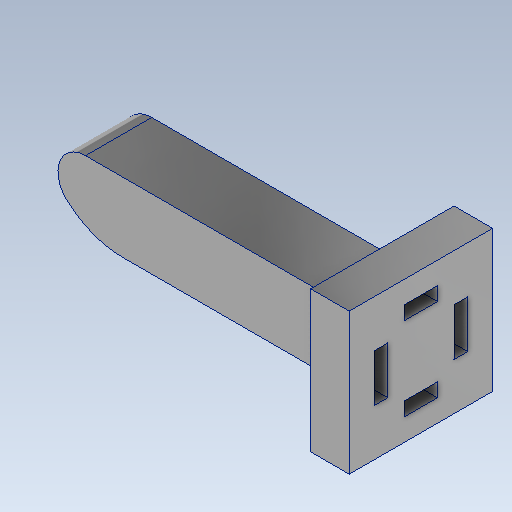
# Autodesk Inventor part: Finray_9_Kerbe_10deg_anschluss_erweitert_9_75 Nut
Saved by Autodesk Inventor 2025.2 (Build 292293000, 293)
## iProperties
Created: 2022-02-28
Part Number: Finray_9_Kerbe_10deg_anschluss_erweitert_9_75 Nut
Material: Generic
Document SubType Name: Modeling
Designer: richa
Density: 1 g/cm^3
Appearance: Aluminum - Flat
Author: richa
## iProperties of the stored document Maria_Greifer_3D-Druck.ipt
Created: 2024-11-10
Part Number: Maria_Greifer_3D-Druck
Material: Generisch
Document SubType Name: Modeling
Designer: maria
Density: 1 g/cm^3
Appearance: Vorgabe
Author: maria
Autodesk Inventor part; units mm, degrees
ref_plane "YZ Plane" through (0, 0, 0) normal (1, 0, 0) x (0, 1, 0)
ref_plane "XZ Plane" through (0, 0, 0) normal (0, 1, 0) x (-1, 0, 0)
ref_plane "XY Plane" through (0, 0, 0) normal (0, 0, 1) x (1, 0, 0)
sketch "Sketch5" plane through (0, 0, 0) normal (0, 0, 1) x (1, 0, 0)
  line L0 (48.5, 0) -> (3.8, 0)
  line L1 (48.5, -12.6) -> (3.8, -12.6)
  line L2 (3.8, -12.6) -> (0, -12.6)
  line L3 (0, -12.6) -> (0, 0)
  line L4 (0, 0) -> (7.8, 0)
  line L5 (38.5, 0) -> (38.5, -12.6)
  line L6 (37.5, -12.6) -> (37.5, 0)
  line L7 (0, -45.1294) -> (0, -34.3361)
  line L8 (0, -34.3361) -> (38.5, -34.3361)
  line L9 (38.5, -34.3361) -> (38.5, -45.1294)
  line L10 (38.5, -45.1294) -> (0, -45.1294)
  line L11 (38.5, -42.4105) -> (39.5, -42.4105)
  line L12 (39.5, -42.4105) -> (39.5, -38.1261)
  line L13 (39.5, -38.1261) -> (38.5, -38.1261)
  line L14 (39.5, -42.4105) -> (39.5, -49.5786)
  line L15 (39.5, -49.5786) -> (45, -49.5786)
  line L16 (45, -49.5786) -> (45, -34.3361)
  line L17 (45, -34.3361) -> (39.5, -34.3361)
  line L18 (39.5, -34.3361) -> (39.5, -38.1261)
  line L19 (48.5, 0) -> (55.8897, 0)
  line L20 (55.8897, 0) -> (55.8897, -12.6)
  line L21 (55.8897, -12.6) -> (48.5, -12.6)
  point P0 (7.8, 0)
  point P1 (39, -42.4105)
  dimension "d63" = 44.7
  dimension "d71" = 0
  dimension "d97" = 12.6
  dimension "d123" = 1
  dimension "d124" = 37.5
  dimension "d125" = 38.5
  dimension "d127" = 1
  dimension "d128" = 5.5
  constraints: 44 end point, 13 perpendicular, 8 point on line, 4 horizontal, 2 vertical, 1 midpoint, 1 parallel
  measures "d63" distance of L1.start L1.end
  measures "d71" distance from line of L3.end L0
  measures "d97" distance of L2.end L3.end
  measures "d123" distance between parallel lines of L5 L6
  measures "d124" distance between parallel lines of L3 L6
  measures "d125" distance of L9.end L7.start
  measures "d127" distance of L11.start L11.end
  measures "d128" distance of L14.end L15.end
extrude "Extrusion2" add sketch "Sketch5" along normal blind 12 contours L19 L20 L21 L1 L5 L0 | L5 L1 L6 L0 | L6 L1 L2 L3 L4 L0
fillet "Fillet2" radius 15 1 edges at (0, -12.6, 6)
fillet "Rundung3" radius 5 1 edges at (0, 0, 6)
sketch "Skizze17" plane through (55.8897, -12.6, 0) normal (1, 0, 0) x (0, 0, -1)
  line L0 (-19, -6.5) -> (7, -6.5)
  line L1 (7, -6.5) -> (7, 19.1)
  line L2 (7, 19.1) -> (-19, 19.1)
  line L3 (-19, 19.1) -> (-19, -6.5)
  line L4 (-19, -6.5) -> (7, 19.1) construction
  line L5 (7, -6.5) -> (-19, 19.1) construction
  line L6 (0, 12.6) -> (-12, 12.6) projected
  line L7 (0, 0) -> (-12, 0) projected
  line L8 (0, 0) -> (0, 12.6) projected
  line L9 (-12, 0) -> (-12, 12.6) projected
  point P0 (-6, 6.3)
  point P1 (7, 6.3)
  dimension "d151" = 26
  dimension "d152" = 25.6
  dimension "d153" = 6.5
  dimension "d154" = 6.5
  dimension "d155" = 7
  dimension "d156" = 7
  constraints: 12 end point, 3 midpoint, 2 parallel, 1 horizontal, 1 perpendicular
  measures "d151" distance of L1.end L2.end
  measures "d152" distance of L2.end L0.start
  measures "d153" distance between parallel lines of L2 L6
  measures "d154" distance between parallel lines of L0 L7
  measures "d155" distance between parallel lines of L3 L9
  measures "d156" distance from line of point (7, 6.3) L8
extrude "Extrusion12" add sketch "Skizze17" along normal blind 7 contours L3 L2 L1 L0 | L8 L7 L9 L6
sketch "Skizze18" plane through (55.8897, -12.6, 0) normal (-1, 0, 0) x (0, 0, 1)
  circle A0 centre (-4.5, 16.6) radius 1.75
  circle A1 centre (16.5, 16.6) radius 1.75
  circle A2 centre (16.5, -4) radius 1.75
  circle A3 centre (-4.5, -4) radius 1.75
  line L0 (-7, 19.1) -> (19, 19.1) projected
  line L1 (-7, -6.5) -> (-7, 19.1) projected
  line L2 (19, 19.1) -> (19, -6.5) projected
  line L3 (19, -6.5) -> (-7, -6.5) projected
  point P0 (0, 12.6)
  dimension "d135" = 3.5
  dimension "d136" = 2.5
  dimension "d137" = 2.5
  dimension "d138" = 3.5
  dimension "d139" = 2.5
  dimension "d140" = 2.5
  dimension "d141" = 2.5
  dimension "d142" = 2.5
  dimension "d143" = 2.5
  dimension "d144" = 2.5
  dimension "d145" = 3.5
  dimension "d146" = 3.5
  constraints: 4 centre point
  measures "d135" diameter of A0
  measures "d136" distance from line of A0.centre L0
  measures "d137" distance from line of L1 A0.centre
  measures "d138" diameter of A1
  measures "d139" distance from line of L0 A1.centre
  measures "d140" distance from line of L2 A1.centre
  measures "d141" distance from line of L3 A2.centre
  measures "d142" distance from line of L2 A2.centre
  measures "d143" distance from line of L1 A3.centre
  measures "d144" distance from line of L3 A3.centre
  measures "d145" diameter of A3
  measures "d146" diameter of A2
extrude "Extrusion13" cut sketch "Skizze18" against normal blind 2.5 contours A0 | A1 | A2 | A3
sketch "Skizze22" plane through (55.8897, -12.6, 0) normal (-1, 0, 0) x (0, 0, 1)
  line L0 (0, 12.6) -> (10, 12.6)
  line L1 (9, 15.1) -> (3, 15.1)
  line L2 (-2.5, 10.6) -> (-2.5, 2)
  line L3 (4.6106, -2.5) -> (9, -2.5)
  line L4 (10, -0.0226) -> (9.9863, -0.0226)
  line L5 (9.9863, 12.8711) -> (10, 12.8711)
  line L6 (14.5, 10.6) -> (14.5, 2)
  line L7 (4.6106, -2.5) -> (3, -2.5)
  line L8 (12, 12.6) -> (0, 12.6) projected
  line L9 (0, 0) -> (0, 12.6) projected
  line L10 (0, 0) -> (0, 12.6)
  line L11 (0, 12.6) -> (12, 12.6)
  line L12 (0, 0) -> (12, 0) projected
  line L13 (0, 0) -> (10, 0)
  line L14 (11.3365, 15.1) -> (11.4, 15.1)
  line L15 (3, 15.1) -> (3, 12.6)
  line L16 (0, 10.6) -> (-2.5, 10.6)
  line L17 (10, 10.6) -> (14.5, 10.6)
  line L18 (9, 12.6) -> (9, 15.1)
  line L19 (0, 2) -> (-2.5, 2)
  line L20 (3, 0) -> (3, -2.5)
  line L21 (9, 0) -> (9, -2.5)
  line L22 (10, 2) -> (14.5, 2)
  line L23 (12, 12.6) -> (12, 3.9) projected
  line L24 (12, 3.9) -> (12, 0) projected
  line L25 (12, 10.6) -> (12, 1.95)
  line L26 (14.5, 2) -> (14.5, 10.6)
  point P0 (9, 13.85)
  point P1 (3, 13.85)
  point P2 (12.25, 2)
  point P3 (12.25, 10.6)
  point P4 (-1.25, 10.6)
  point P5 (-1.25, 2)
  point P6 (3, 0)
  point P7 (0, 2)
  point P8 (3, 12.6)
  point P9 (9, 12.6)
  point P10 (14.5, 6.3)
  point P11 (12, 2)
  dimension "d172" = 0
  dimension "d173" = 2.5
  dimension "d175" = 2.5
  dimension "d176" = 2.5
  dimension "d180" = 3
  dimension "d181" = 3
  dimension "d183" = 2
  dimension "d184" = 2
  dimension "d185" = 2
  dimension "d186" = 2
  dimension "d190" = 2.5
  dimension "d191" = 3
  dimension "d192" = 3
  constraints: 44 end point, 13 point on line, 8 midpoint, 5 perpendicular, 4 collinear, 4 horizontal, 3 parallel
  measures "d172" distance between parallel lines of L0 L8
  measures "d173" distance between parallel lines of L0 L1
  measures "d175" distance between parallel lines of L9 L2
  measures "d176" distance from line of L3.start L12
  measures "d180" distance from line of L9 point (3, 13.85)
  measures "d181" distance between parallel lines of L9 L20
  measures "d183" distance from line of L12 point (12.25, 2)
  measures "d184" distance from line of L0 point (12.25, 10.6)
  measures "d185" distance from line of point (-1.25, 10.6) L0
  measures "d186" distance from line of L12 point (-1.25, 2)
  measures "d190" distance from line of L23 point (14.5, 6.3)
  measures "d191" distance from line of L21.start L24
  measures "d192" distance between parallel lines of L18 L23
extrude "Extrusion19" cut sketch "Skizze22" against normal blind 10 contours L15 L1 L18 L0 | L9 L19 L2 L16 | L12 L21 L3 L7 L20 | L17 L6 L22 L24 L23
equation "\"l1\" = 8"
body "Solid2"
